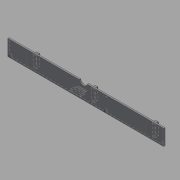
# Autodesk Inventor part: xtion_mainboard
Saved by Autodesk Inventor 2017 (Build 210142000, 142)
## iProperties
Created: 2016-11-18
Part Number: xtion_mainboard
Material: Generic
Document SubType Name: Modeling
Designer: Ali
Density: 1 g/cm^3
Appearance: Default
Author: Ali
Autodesk Inventor part; units mm, degrees
ref_plane "YZ Plane" through (0, 0, 0) normal (1, 0, 0) x (0, 1, 0)
ref_plane "XZ Plane" through (0, 0, 0) normal (0, 1, 0) x (-1, 0, 0)
ref_plane "XY Plane" through (0, 0, 0) normal (0, 0, 1) x (1, 0, 0)
sketch "Sketch1" plane through (0, 0, 0) normal (0, 1, 0) x (-1, 0, 0)
  line L0 (79, -8) -> (-79, -8)
  line L1 (-79, -8) -> (-79, 8)
  line L2 (79, 8) -> (79, -8)
  line L3 (79, -8) -> (-79, 8) construction
  line L4 (-79, -8) -> (79, 8) construction
  arc A0 (-1.6, 8) -> (6.6, 8) centre (2.5, 9.0266) ccw
  line L5 (0, -8) -> (0, 2.5887)
  line L6 (2.5, 9.0266) -> (2.5, 15.2917) construction
  line L7 (7.7992, 4.8) -> (-2.6665, 4.8) construction
  line L8 (-79, 8) -> (-1.6, 8)
  line L9 (6.6, 8) -> (79, 8)
  point P0 (0, 0)
  dimension "d0" = 158
  dimension "d1" = 16
  dimension "d2" = 76.5
  dimension "d3" = 8.2
  dimension "d5" = 3.2
  constraints: 20 end point, 3 midpoint, 3 parallel, 2 horizontal, 2 point on circle, 2 vertical, 1 centre point, 1 collinear, 1 perpendicular, 1 tangent
  measures "d0" distance of L1.end L2.start
  measures "d1" distance of L0.end L1.end
  measures "d2" distance between parallel lines of L2 L6
  measures "d3" distance of L8.end L9.start
  measures "d5" distance between parallel lines of L9 L7
extrude "Extrusion1" add sketch "Sketch1" along normal blind 1.3
sketch "Sketch2" plane through (0, 1.3, 0) normal (0, 1, 0) x (1, 0, 0)
  line L0 (79, 8) -> (-79, 8) projected
  line L1 (-79, 8) -> (-79, -8) projected
  line L2 (-79, -8) -> (-6.6, -8) projected
  arc A0 (1.6, -8) -> (-6.6, -8) centre (-2.5, -9.0266) ccw projected
  line L3 (1.6, -8) -> (79, -8) projected
  line L4 (79, -8) -> (79, 8) projected
  line L5 (-77, 6.2) -> (77, 6.2) construction
  line L6 (19.5, 6.2) -> (19.5, -6.2) construction
  point P0 (0, 0)
  dimension "d8" = 154
  dimension "d9" = 1.8
  dimension "d10" = 1.8
  dimension "d11" = 57.5
  dimension "d19" = 2
  dimension "d20" = 2
  dimension "d47" = 59.5
  constraints: 4 end point, 1 horizontal, 1 point on line, 1 vertical
  measures "d8" distance of L5.start L5.end
  measures "d9" distance from line of L0 L5.end
  measures "d10" distance from line of L3 L6.end
  measures "d11" distance of L5.end L6.start
  measures "d19" distance from line of L1 L5.start
  measures "d20" distance from line of L4 L5.end
  measures "d47" distance from line of L6.end L4
hole "Hole1" at (-77, 1.3, -6.2) at (77, 1.3, -6.2) at (19.5, 1.3, -6.2) at (19.5, 1.3, 6.2) direction (0, -1, 0) diameter 1.9 end through all
sketch "Sketch3" plane through (0, 1.3, 0) normal (0, 1, 0) x (1, 0, 0)
  line L0 (-16.35, 7.5) -> (-6.5, 7.5)
  line L1 (-6.5, 7.5) -> (-6.5, 5.5)
  line L2 (-6.5, 5.5) -> (-16.35, 5.5)
  line L3 (-16.35, 5.5) -> (-16.35, 7.5)
  line L4 (-16.35, 7.5) -> (-6.5, 5.5) construction
  line L5 (-6.5, 7.5) -> (-16.35, 5.5) construction
  line L6 (79, 8) -> (-79, 8) projected
  line L7 (-79, 8) -> (-79, -8) projected
  line L8 (-54.7, -5.85) -> (-51.7, -5.85)
  line L9 (-51.7, -5.85) -> (-51.7, 5.85)
  line L10 (-51.7, 5.85) -> (-54.7, 5.85)
  line L11 (-54.7, 5.85) -> (-54.7, -5.85)
  line L12 (-54.7, -5.85) -> (-51.7, 5.85) construction
  line L13 (-51.7, -5.85) -> (-54.7, 5.85) construction
  line L14 (4.6, -6.1) -> (7.4, -6.1)
  line L15 (7.4, -6.1) -> (7.4, 6.1)
  line L16 (7.4, 6.1) -> (4.6, 6.1)
  line L17 (4.6, 6.1) -> (4.6, -6.1)
  line L18 (4.6, -6.1) -> (7.4, 6.1) construction
  line L19 (7.4, -6.1) -> (4.6, 6.1) construction
  line L20 (66, -6.1) -> (68.8, -6.1)
  line L21 (68.8, -6.1) -> (68.8, 6.1)
  line L22 (68.8, 6.1) -> (66, 6.1)
  line L23 (66, 6.1) -> (66, -6.1)
  line L24 (66, -6.1) -> (68.8, 6.1) construction
  line L25 (68.8, -6.1) -> (66, 6.1) construction
  line L26 (6, 0) -> (67.4, 0) construction
  line L27 (79, -8) -> (79, 8) projected
  point P0 (0, 0)
  point P1 (-11.425, 6.5)
  point P2 (-53.2, 0)
  point P3 (-53.2, 0)
  dimension "d21" = 9.85
  dimension "d22" = 2
  dimension "d23" = 0.5
  dimension "d24" = 72.5
  dimension "d25" = 3
  dimension "d26" = 11.7
  dimension "d27" = 2.8
  dimension "d28" = 12.2
  dimension "d29" = 12.2
  dimension "d30" = 2.8
  dimension "d31" = 74.4
  dimension "d32" = 13
  dimension "d33" = 27.3
  constraints: 50 end point, 9 midpoint, 8 parallel, 4 horizontal, 4 perpendicular, 3 point on line
  measures "d21" distance of L1.end L2.end
  measures "d22" distance of L0.end L1.end
  measures "d23" distance between parallel lines of L0 L6
  measures "d24" distance between parallel lines of L1 L7
  measures "d25" distance of L9.end L10.end
  measures "d26" distance of L8.end L9.end
  measures "d27" distance of L15.end L16.end
  measures "d28" distance of L14.end L15.end
  measures "d29" distance of L20.end L21.end
  measures "d30" distance of L21.end L22.end
  measures "d31" distance between parallel lines of L27 L17
  measures "d32" distance between parallel lines of L27 L23
  measures "d33" distance between parallel lines of L9 L7
extrude "Extrusion2" add sketch "Sketch3" along normal blind 3.6
sketch "Sketch4" plane through (0, 4.9, 0) normal (0, 1, 0) x (1, 0, 0)
  line L0 (-6.5, 7.5) -> (-16.35, 7.5) projected
  line L1 (-16.35, 7.5) -> (-16.35, 5.5) projected
  line L2 (-16.35, 5.5) -> (-6.5, 5.5) projected
  line L3 (-6.5, 5.5) -> (-6.5, 7.5) projected
  line L4 (-16.35, 6.5) -> (-6.5, 6.5) construction
  line L5 (-6.5, 7.5) -> (-6.5, 5.5) projected
  circle A0 centre (-15.375, 6.5) radius 0.25
  circle A1 centre (-7.475, 6.5) radius 0.25
  circle A2 centre (-13.4, 6.5) radius 0.25
  circle A3 centre (-11.425, 6.5) radius 0.25
  circle A4 centre (-9.45, 6.5) radius 0.25
  line L6 (-6.5, 5.5) -> (-16.35, 5.5) projected
  line L7 (-11.425, 5.5) -> (-11.425, 4.6298) construction
  point P0 (0, 0)
  dimension "d36" = 0.5
  dimension "d37" = 0.5
  dimension "d38" = 7.9
  dimension "d39" = 0.5
  dimension "d40" = 0.5
  dimension "d41" = 0.5
  dimension "d42" = 1.975
  dimension "d43" = 1.975
  dimension "d44" = 1.975
  constraints: 5 centre point, 5 point on line, 4 end point, 4 midpoint, 1 vertical
  measures "d36" diameter of A0
  measures "d37" diameter of A1
  measures "d38" distance of A1.centre A0.centre
  measures "d39" diameter of A2
  measures "d40" diameter of A3
  measures "d41" diameter of A4
  measures "d42" distance of A2.centre A0.centre
  measures "d43" distance of A3.centre A2.centre
  measures "d44" distance of A4.centre A3.centre
extrude "Extrusion3" add sketch "Sketch4" along normal blind 3.6 contours A0 | A1 | A2 | A3 | A4
equation "\"d10\" = d9"
equation "\"d29\" = d28"
equation "\"d30\" = d27"
equation "\"d42\" = 0.25 * d38"
equation "\"d43\" = d42"
equation "\"d44\" = d43"
body "Solid1"
